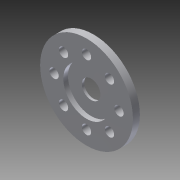
# Autodesk Inventor part: 13
Saved by Autodesk Inventor 2013 (Build 170138000, 138)
## iProperties
Created: 2014-03-29
Part Number: 13
Material: アセタール樹脂、白
Document SubType Name: Modeling
Designer: andou
Density: 1 g/cm^3
Author: andou
Title: Horn-Spacer
Autodesk Inventor part; units mm, degrees
ref_plane "YZ Plane" through (0, 0, 0) normal (1, 0, 0) x (0, 1, 0)
ref_plane "XZ Plane" through (0, 0, 0) normal (0, 1, 0) x (-1, 0, 0)
ref_plane "XY Plane" through (0, 0, 0) normal (0, 0, 1) x (1, 0, 0)
sketch "スケッチ1" plane through (0, 0, 0) normal (0, 1, 0) x (-1, 0, 0)
  circle A0 centre (0, 0) radius 10
  dimension "d0" = 20
  constraints: 1 centre point, 1 coincident
  measures "d0" diameter of A0
extrude "押し出し2" add sketch "スケッチ1" along normal blind 1.5
sketch "スケッチ3" plane through (0, 0, 0) normal (0, -1, 0) x (1, 0, 0)
  circle A0 centre (0, 0) radius 10 projected
  circle A1 centre (0, 0) radius 2
  dimension "d21" = 4
  constraints: 1 centre point, 1 coincident
  measures "d21" diameter of A1
hole "穴2" at (0, 0, 0) direction (0, 1, 0) diameter 4 end through all counterbore diameter 10 counterbore depth 1
sketch "スケッチ4" plane through (0, 0, 0) normal (0, -1, 0) x (1, 0, 0)
  circle A0 centre (0, 0) radius 5 projected
  circle A1 centre (0, 7) radius 1
  dimension "d30" = 0
  dimension "d31" = 7
  dimension "d32" = 2
  constraints: 1 centre point
  measures "d30" horizontal distance of A1.centre A0.centre
  measures "d31" distance of A0.centre A1.centre
  measures "d32" diameter of A1
hole "穴3" at (0, 0, 7) direction (0, 1, 0) diameter 2 end through all
pattern_circular "円形状パターン2" count 8 over 360 about axis through (0, 0.5, 0) along (0, -1, 0) of "穴3"
